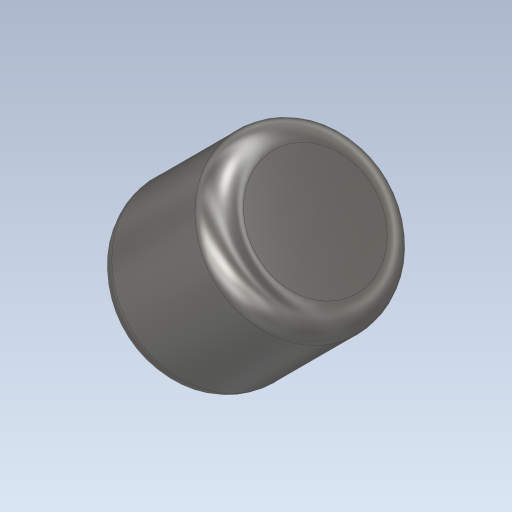
# Autodesk Inventor part: CRBT155A_PART3
Saved by Autodesk Inventor 2024 (Build 280153000, 153)
## iProperties
Created: 2023-09-04
Part Number: CRBT155A_PART3
Material: ステンレス鋼
Catalog Web Link: www.cadenas.de
Description: -
Vendor: IKO
Document SubType Name: Modeling
Designer: psAdmin
Manufacturer: IKO
Mass: 0.0484539 g
Surface Area: 0.171514 cm^2
Volume: 0.00605674 cm^3
Density: 8 g/cm^3
Appearance: 半つや出し
Category: PARTsolutions
Company: IKO
PSOL_IDENT_0: {$CADENAS_DATA/23d-libs/iko/iko_bearings/crossed_rb/ultra_slim_type_crb/ultra_slim_type_crbt.prj},23
PSOL_IDENT_1: 2 {VTYP=3D},{NB=CRBT155A_PART3},{LINA=CRBT155A_PART3},{NN=Ultra Slim Type Crossed Roller Bearings (C
PSOL_IDENT_2: RBT...A)_PART3},{NOPRJ=TRUE},{DATE=09.07.2020 23:28:49},{GEOMDATE=08.07.2020 06:24:28},{VERSION=},{L
PSOL_IDENT_3: INEID=220},{WBVAR=},{WBNUMERIC=}  {NB=CRBT155A_PART3},{LINA=CRBT155A_PART3},{KT=DUMMY},{IDNR=},{STDR
PSOL_IDENT_4: T=15},{ORDER=CRBT155A},{MASS=11.9},{SD=15},{D=26},{B=5},{SR=0.15},{SDA=17.5},{DA=22.0},{DAR=2.0},{ZE
PSOL_IDENT_5: FF=16},{RS=0.3},{DETC=1.6},{PCDRL=19.6},{SDOR=20.10},{DIRR=19.10},{COG=0.0},{SDOG=0.0},{OH=0.0},{NH=
PSOL_IDENT_6: 0},{CR=1320},{COR=1110},{SC=0},{N=8},{N1=1.67}
NB: CRBT155A_PART3
NBSYN: $ORDER._PART3
LINA: CRBT155A_PART3
CATALOG: IKO (Nippon Thompson
STDRT: 15
ORDER: CRBT155A
MASS: 11.9
SD: 15
D: 26
B: 5
SR: 0.15
SDA: 17.5
DA: 22
CR: 1320
COR: 1110
SUPPLIER: IKO
ARTICLENO: CRBT155A_PART3
BOMINFO: CRBT155A_PART3
CREATOR: CADENAS GmbH
Title: CRBT155A_PART3
Author: Cadenas PARTsolutions
Autodesk Inventor part; units mm, degrees
ref_plane "YZ Plane" through (0, 0, 0) normal (1, 0, 0) x (0, 1, 0)
ref_plane "XZ Plane" through (0, 0, 0) normal (0, 1, 0) x (-1, 0, 0)
ref_plane "XY Plane" through (0, 0, 0) normal (0, 0, 1) x (1, 0, 0)
sketch "Sketch_1" plane through (0, 0, 0) normal (0, 0, 1) x (1, 0, 0)
  line L0 (1.7929, 9.0929) -> (3.2071, 10.5071)
  line L1 (3.2071, 10.5071) -> (3.7021, 10.0121)
  arc A0 (3.7021, 9.5879) -> (3.7021, 10.0121) centre (3.4899, 9.8) ccw
  line L2 (3.7021, 9.5879) -> (2.7121, 8.5979)
  arc A1 (2.2879, 8.5979) -> (2.7121, 8.5979) centre (2.5, 8.8101) ccw
  line L3 (2.2879, 8.5979) -> (1.7929, 9.0929)
  line L4 (1.7929, 9.0929) -> (3.2071, 10.5071)
  constraints: 10 end point, 4 point on circle, 2 centre point
revolve "Revolution1" add sketch "Sketch_1" angle 360 about axis through (1.7929, 9.0929, 0) along (-0.7071, -0.7071, 0)
body "Solid1"
